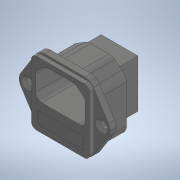
# Autodesk Inventor part: IEC Receptacle
Saved by Autodesk Inventor 2020 (Build 240168000, 168)
## iProperties
Created: 2019-06-19
Part Number: IEC Receptacle
Material: ABS Plastic
Document SubType Name: Modeling
Designer: pepd9
Density: 1.06 g/cm^3
Appearance: Gray
Author: pepd9
Autodesk Inventor part; units mm, degrees
ref_plane "YZ Plane" through (0, 0, 0) normal (1, 0, 0) x (0, 1, 0)
ref_plane "XZ Plane" through (0, 0, 0) normal (0, 1, 0) x (-1, 0, 0)
ref_plane "XY Plane" through (0, 0, 0) normal (0, 0, 1) x (1, 0, 0)
sketch "Sketch1" plane through (0, 0, 0) normal (0, 0, 1) x (1, 0, 0)
  line L0 (-14.1, -15.5) -> (14.1, -15.5)
  line L1 (14.1, -15.5) -> (14.1, 15.5)
  line L2 (14.1, 15.5) -> (-14.1, 15.5)
  line L3 (-14.1, 15.5) -> (-14.1, -15.5)
  line L4 (-14.1, -15.5) -> (14.1, 15.5) construction
  line L5 (14.1, -15.5) -> (-14.1, 15.5) construction
  point P0 (0, 0)
  dimension "d0" = 28.2
  dimension "d1" = 31
  constraints: 12 end point, 2 midpoint, 2 parallel, 1 horizontal, 1 perpendicular
  measures "d0" distance of L2.end L1.end
  measures "d1" distance of L1.end L0.end
extrude "Extrusion1" add sketch "Sketch1" along normal blind 2
fillet "Fillet1" radius 2.5 4 edges at (-14.1, 15.5, 1) (14.1, 15.5, 1) (14.1, -15.5, 1) (-14.1, -15.5, 1)
sketch "Sketch2" plane through (0, 0, 0) normal (0, 0, -1) x (-1, 0, 0)
  line L0 (-22, -16.5) -> (22, -16.5)
  line L1 (22, -16.5) -> (22, 16.5)
  line L2 (22, 16.5) -> (-22, 16.5)
  line L3 (-22, 16.5) -> (-22, -16.5)
  line L4 (-22, -16.5) -> (22, 16.5) construction
  line L5 (22, -16.5) -> (-22, 16.5) construction
  point P0 (0, 0)
  dimension "d5" = 44
  dimension "d6" = 33
  constraints: 12 end point, 2 midpoint, 2 parallel, 1 horizontal, 1 perpendicular
  measures "d5" distance of L2.end L1.end
  measures "d6" distance of L1.end L0.end
extrude "Extrusion2" add sketch "Sketch2" along normal blind 3
chamfer "Chamfer1" distance 9.5 distance2 15 1 edges at (22, 16.5, -1.5) measured on face at (21.5, 16.5, -1.5)
chamfer "Chamfer2" distance 9.5 distance2 15 1 edges at (22, -16.5, -1.5) measured on face at (21.5, -16.5, -1.5)
chamfer "Chamfer3" distance 9.5 distance2 15 1 edges at (-22, -16.5, -1.5) measured on face at (-21.5, -16.5, -1.5)
chamfer "Chamfer4" distance 9.5 distance2 15 1 edges at (-22, 16.5, -1.5) measured on face at (-21.5, 16.5, -1.5)
fillet "Fillet2" radius 5 8 edges at (-12.5, 16.5, -1.5) (-22, 1.5, -1.5) (-22, -1.5, -1.5) (-12.5, -16.5, -1.5) (12.5, -16.5, -1.5) (22, -1.5, -1.5) (22, 1.5, -1.5) (12.5, 16.5, -1.5)
sketch "Sketch3" plane through (0, 0, 0) normal (0, 0, 1) x (1, 0, 0)
  point P0 (0, 0)
  point P1 (-18, 0)
  point P2 (18, 0)
  dimension "d22" = 36
  dimension "d23" = 18
  measures "d22" distance of point (-18, 0) point (18, 0)
  measures "d23" distance of point (0, 0) point (-18, 0)
hole "Hole1" at (-18, 0, 0) at (18, 0, 0) direction (0, 0, -1) diameter 3.4 end through all countersink diameter 6 countersink angle 90
sketch "Sketch4" plane through (0, 0, 2) normal (0, 0, 1) x (1, 0, 0)
  line L0 (11, -6.8281) -> (-11, -6.8281)
  line L1 (-11, -6.8281) -> (-11, -12.8281)
  line L2 (-11, -12.8281) -> (11, -12.8281)
  line L3 (11, -12.8281) -> (11, -6.8281)
  line L4 (11, -6.8281) -> (-11, -12.8281) construction
  line L5 (-11, -6.8281) -> (11, -12.8281) construction
  point P0 (0, 0)
  point P1 (0, -9.8281)
  dimension "d31" = 22
  dimension "d32" = 6
  constraints: 12 end point, 2 midpoint, 2 parallel, 1 horizontal, 1 perpendicular
  measures "d31" distance of L2.end L1.end
  measures "d32" distance of L1.end L0.end
extrude "Extrusion3" cut sketch "Sketch4" against normal blind 0.2
sketch "Sketch5" plane through (0, 0, 2) normal (0, 0, 1) x (1, 0, 0)
  line L0 (-12, 13.3) -> (12, 13.3)
  line L1 (12, 13.3) -> (12, -2.7)
  line L2 (12, -2.7) -> (-12, -2.7)
  line L3 (-12, -2.7) -> (-12, 13.3)
  line L4 (-12, 13.3) -> (12, -2.7) construction
  line L5 (12, 13.3) -> (-12, -2.7) construction
  line L6 (-9.7482, 16.5) -> (9.7482, 16.5) projected
  line L7 (-12, 9.3) -> (-7, 13.3)
  line L8 (7, 13.3) -> (12, 9.3)
  point P0 (0, 0)
  point P1 (0, 5.3)
  dimension "d35" = 24
  dimension "d36" = 16
  dimension "d37" = 3.2
  dimension "d38" = 12
  dimension "d53" = 5
  dimension "d54" = 5
  dimension "d55" = 4
  dimension "d56" = 4
  constraints: 16 end point, 4 point on line, 2 midpoint, 2 parallel, 1 horizontal, 1 perpendicular
  measures "d35" distance of L1.end L2.end
  measures "d36" distance of L0.end L1.end
  measures "d37" distance between parallel lines of L6 L0
  measures "d38" distance from line of point (0, 0) L1
  measures "d53" distance from line of L1 L8.start
  measures "d54" distance from line of L3 L7.end
  measures "d55" distance of L0.start L7.start
  measures "d56" distance of L0.end L8.end
sketch "Sketch6" plane through (0, 0, -3) normal (0, 0, -1) x (-1, 0, 0)
  line L0 (-13.4, -15.4) -> (13.4, -15.4)
  line L1 (13.4, -15.4) -> (13.4, 15.4)
  line L2 (13.4, 15.4) -> (-13.4, 15.4)
  line L3 (-13.4, 15.4) -> (-13.4, -15.4)
  line L4 (-13.4, -15.4) -> (13.4, 15.4) construction
  line L5 (13.4, -15.4) -> (-13.4, 15.4) construction
  point P0 (0, 0)
  dimension "d39" = 26.8
  dimension "d40" = 30.8
  constraints: 12 end point, 2 midpoint, 2 parallel, 1 horizontal, 1 perpendicular
  measures "d39" distance of L2.end L1.end
  measures "d40" distance of L1.end L0.end
extrude "Extrusion4" add sketch "Sketch6" along normal blind 13.6
chamfer "Chamfer5" distance 5 distance2 8 1 edges at (-13.4, 15.4, -9.8) measured on face at (-13.4, 14.9, -9.8)
chamfer "Chamfer6" distance 7 distance2 5 1 edges at (13.4, 15.4, -9.8) measured on face at (12.9, 15.4, -9.8)
fillet "Fillet3" radius 5 6 edges at (-5.4, 15.4, -9.8) (-13.4, 10.4, -9.8) (-13.4, -15.4, -9.8) (13.4, -15.4, -9.8) (13.4, 10.4, -9.8) (6.4, 15.4, -9.8)
sketch "Sketch7" plane through (0, 0, -16.6) normal (0, 0, -1) x (-1, 0, 0)
  line L0 (-8.9018, 11.6252) -> (8.9018, 11.6252)
  line L1 (8.9018, 11.6252) -> (8.9018, -11.6252)
  line L2 (8.9018, -11.6252) -> (-8.9018, -11.6252)
  line L3 (-8.9018, -11.6252) -> (-8.9018, 11.6252)
  line L4 (-8.9018, 11.6252) -> (8.9018, -11.6252) construction
  line L5 (8.9018, 11.6252) -> (-8.9018, -11.6252) construction
  line L6 (7.9018, -10.6252) -> (7.9018, 10.6252)
  line L7 (7.9018, 10.6252) -> (-7.9018, 10.6252)
  line L8 (-7.9018, 10.6252) -> (-7.9018, -10.6252)
  line L9 (-7.9018, -10.6252) -> (7.9018, -10.6252)
  point P0 (0, 0)
  dimension "d50" = 1
  constraints: 20 end point, 4 parallel, 2 midpoint, 2 perpendicular, 1 horizontal, 3 other
  measures "d50" distance between parallel lines of L1 L6
extrude "Extrusion5" add sketch "Sketch7" along normal blind 10
extrude "Extrusion6" cut sketch "Sketch5" against normal blind 16 contours L0 L8 L1 L2 L3 L7
fillet "Fillet4" radius 3 6 edges at (-12, -2.7, -6) (12, -2.7, -6) (12, 9.3, -6) (7, 13.3, -6) (-7, 13.3, -6) (-12, 9.3, -6)
body "Solid1"
